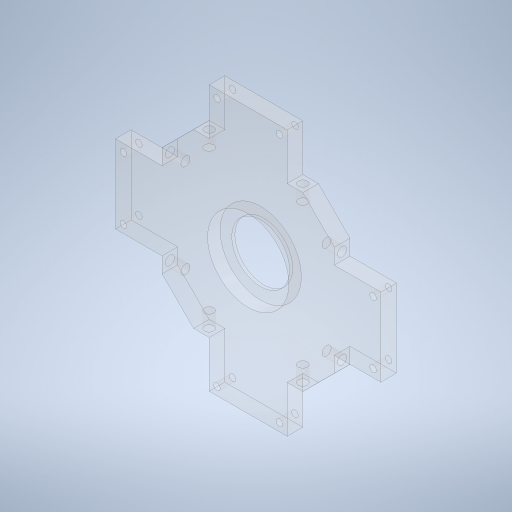
# Autodesk Inventor part: gearbox_base
Saved by Autodesk Inventor 2023 (Build 270158000, 158)
## iProperties
Created: 2023-05-27
Part Number: gearbox_base
Material: PMMA Plastic
Document SubType Name: Modeling
Designer: 310611102
Density: 1.188 g/cm^3
Appearance: Polycarbonate - Clear
Vendor: 新采硯
Author: 310611102
Autodesk Inventor part; units mm, degrees
ref_plane "YZ Plane" through (0, 0, 0) normal (1, 0, 0) x (0, 1, 0)
ref_plane "XZ Plane" through (0, 0, 0) normal (0, 1, 0) x (-1, 0, 0)
ref_plane "XY Plane" through (0, 0, 0) normal (0, 0, 1) x (1, 0, 0)
sketch "Sketch1" plane through (0, 0, 0) normal (0, 0, 1) x (1, 0, 0)
  line L0 (-25, 65.19) -> (25, 65.19)
  line L1 (65.19, 25) -> (65.19, -25)
  line L2 (25, -65.19) -> (-25, -65.19)
  line L3 (-65.19, -25) -> (-65.19, 25)
  line L4 (-50.6308, 50.6308) -> (50.6308, -50.6308) construction
  line L5 (50, 50) -> (-50, -50) construction
  line L6 (-40, 40) -> (-50.6308, 50.6308) construction
  line L7 (-25, 65.19) -> (-25, 55.19)
  line L8 (-25, 55.19) -> (-35, 55.19)
  line L9 (-55.19, 35) -> (-55.19, 25)
  line L10 (-55.19, 25) -> (-65.19, 25)
  circle A0 centre (0, 0) radius 26
  line L11 (0, 28.0827) -> (0, 0)
  line L12 (0, 0) -> (17.6422, 0)
  line L13 (25, 65.19) -> (25, 55.19)
  line L14 (25, 55.19) -> (35, 55.19)
  line L15 (55.19, 35) -> (55.19, 25)
  line L16 (55.19, 25) -> (65.19, 25)
  line L17 (-25, -65.19) -> (-25, -55.19)
  line L18 (-25, -55.19) -> (-35, -55.19)
  line L19 (-55.19, -35) -> (-55.19, -25)
  line L20 (-55.19, -25) -> (-65.19, -25)
  line L21 (25, -65.19) -> (25, -55.19)
  line L22 (25, -55.19) -> (35, -55.19)
  line L23 (55.19, -35) -> (55.19, -25)
  line L24 (55.19, -25) -> (65.19, -25)
  line L25 (-35, 55.19) -> (-55.19, 35)
  line L26 (35, 55.19) -> (55.19, 35)
  line L27 (55.19, -35) -> (35, -55.19)
  line L28 (-35, -55.19) -> (-55.19, -35)
  point P0 (-45.3154, 45.3154)
  point P1 (-55.19, 55.19)
  point P2 (55.19, 55.19)
  point P3 (-55.19, -55.19)
  point P4 (55.19, -55.19)
  dimension "d9" = 130.38
  dimension "d19" = 10
  dimension "d20" = 52
  dimension "d40" = 130.38
  dimension "d45" = 10
  dimension "d58" = 50
  dimension "d59" = 50
  dimension "d60" = 20.19
  dimension "d61" = 20.19
  dimension "d62" = 20.19
  dimension "d63" = 20.19
  dimension "d64" = 20.19
  dimension "d65" = 20.19
  dimension "d66" = 20.19
  dimension "d67" = 20.19
  dimension "d79" = 10
  constraints: 58 end point, 13 symmetric about line, 9 point on line, 5 perpendicular, 3 midpoint, 3 vertical, 2 horizontal, 2 parallel, 1 centre point, 1 coincident
  measures "d9" distance between parallel lines of L2 L0
  measures "d19" distance of L0.start L7.end
  measures "d20" diameter of A0
  measures "d40" distance between parallel lines of L1 L3
  measures "d45" distance of L9.end L3.end
  measures "d58" distance of L0.start L0.end
  measures "d59" distance of L3.start L3.end
  measures "d60" distance of L8.end point (-55.19, 55.19)
  measures "d61" distance of L9.start point (-55.19, 55.19)
  measures "d62" distance of L14.end point (55.19, 55.19)
  measures "d63" distance of L15.start point (55.19, 55.19)
  measures "d64" distance of L23.start point (55.19, -55.19)
  measures "d65" distance of L22.end point (55.19, -55.19)
  measures "d66" distance of L18.end point (-55.19, -55.19)
  measures "d67" distance of L19.start point (-55.19, -55.19)
  measures "d79" distance of L7.end L8.end
extrude "Extrusion1" add sketch "Sketch1" along normal blind 10
sketch "Sketch3" plane through (0, 0, 10) normal (0, 0, 1) x (1, 0, 0)
  line L0 (25, 65.19) -> (-25, 65.19) projected
  line L1 (25, 65.19) -> (-25, 65.19)
  line L2 (-25, 65.19) -> (-25, 85)
  line L3 (-25, 85) -> (25, 85)
  line L4 (25, 85) -> (25, 65.19)
  line L5 (-25, 65.19) -> (-25, 55.19) projected
  circle A0 centre (-20, 80) radius 2.1
  line L6 (0, 0) -> (0, 7.5781)
  circle A1 centre (20, 80) radius 2.1
  circle A2 centre (-80, -20) radius 2.1
  circle A3 centre (-80, 20) radius 2.1
  circle A4 centre (20, -80) radius 2.1
  circle A5 centre (-20, -80) radius 2.1
  circle A6 centre (80, 20) radius 2.1
  circle A7 centre (80, -20) radius 2.1
  line L7 (25, 55.19) -> (25, 65.19) projected
  line L8 (-65.19, 25) -> (-65.19, -25)
  line L9 (-85, 25) -> (-65.19, 25)
  line L10 (-85, -25) -> (-85, 25)
  line L11 (-65.19, -25) -> (-85, -25)
  line L12 (-25, -65.19) -> (25, -65.19)
  line L13 (-25, -85) -> (-25, -65.19)
  line L14 (25, -85) -> (-25, -85)
  line L15 (25, -65.19) -> (25, -85)
  line L16 (65.19, -25) -> (65.19, 25)
  line L17 (85, -25) -> (65.19, -25)
  line L18 (85, 25) -> (85, -25)
  line L19 (65.19, 25) -> (85, 25)
  point P0 (-25, 60.19)
  point P1 (-25, 75.095)
  point P2 (-75.095, -25)
  point P3 (25, -75.095)
  point P4 (75.095, 25)
  dimension "d31" = 4.2
  dimension "d35" = 360
  dimension "d43" = 360
  dimension "d49" = 5
  dimension "d50" = 40
  dimension "d51" = 5
  dimension "d80" = 170
  constraints: 34 end point, 8 centre point, 4 point on line, 2 midpoint, 2 parallel, 1 collinear, 1 horizontal, 1 perpendicular, 1 symmetric about line, 1 vertical, 1 vertical alignment, 59 other
  measures "d31" diameter of A0
  measures "d49" distance from line of L2 A0.centre
  measures "d50" distance of A1.centre A0.centre
  measures "d51" distance from line of L3 A0.centre
  measures "d80" distance between parallel lines of L14 L3
extrude "Extrusion3" add sketch "Sketch3" against normal up to surface (10 mm away)
sketch "Sketch5" plane through (0, 0, 0) normal (0, 0, -1) x (-1, 0, 0)
  circle A0 centre (0, 0) radius 26 projected
  circle A1 centre (0, 0) radius 18.5
  dimension "d55" = 37
  constraints: 1 centre point, 1 coincident
  measures "d55" diameter of A1
extrude "Extrusion5" add sketch "Sketch5" against normal blind 2
sketch "Sketch6" plane through (-35, 55.19, 0) normal (0, 1, 0) x (1, 0, 0)
  circle A0 centre (5, -5) radius 2.9
  line L0 (10, -10) -> (0, -10) projected
  line L1 (10, -10) -> (10, 0) projected
  point P0 (35, 0)
  dimension "d68" = 5
  dimension "d69" = 5
  dimension "d70" = 5.8
  constraints: 1 centre point
  measures "d68" distance from line of L0 A0.centre
  measures "d69" distance from line of L1 A0.centre
  measures "d70" diameter of A0
extrude "Extrusion6" cut sketch "Sketch6" against normal blind 10
mirror "Mirror1" about plane through (0, 0, 0) normal (1, 0, 0) of "Extrusion6"
pattern_circular "Circular Pattern2" count 4 over 360 about axis through (0, 0, 0) along (0, 0, 1) of "Extrusion6", "Mirror1"
equation "\"d9\" = d40"
equation "\"d59\" = d58"
equation "\"d61\" = d60"
equation "\"d62\" = d60"
equation "\"d63\" = d62"
equation "\"d64\" = d60"
equation "\"d65\" = d64"
equation "\"d66\" = d60"
equation "\"d67\" = d66"
body "Solid1"
